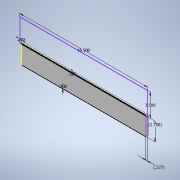
# Autodesk Inventor part: Part3
Saved by Autodesk Inventor 2021 (Build 250183000, 183)
## iProperties
Created: 2020-09-03
Part Number: Part3
Material: Generic
Document SubType Name: Modeling
Designer: deli
Density: 1 g/cm^3
Appearance: Default
Author: deli
Autodesk Inventor part; units mm, degrees
ref_plane "YZ Plane" through (0, 0, 0) normal (1, 0, 0) x (0, 1, 0)
ref_plane "XZ Plane" through (0, 0, 0) normal (0, 1, 0) x (-1, 0, 0)
ref_plane "XY Plane" through (0, 0, 0) normal (0, 0, 1) x (1, 0, 0)
sketch "Sketch1" plane through (0, 0, 0) normal (0, 0, 1) x (1, 0, 0)
  line L0 (-47.5672, 9.4536) -> (435.0328, 9.4536)
  line L1 (435.0328, 9.4536) -> (435.0328, -60.3964)
  line L2 (435.0328, -60.3964) -> (-47.5672, -60.3964)
  line L3 (-47.5672, -60.3964) -> (-47.5672, 9.4536)
  point P0 (0, 0)
  dimension "d0" = 482.6
  dimension "d1" = 69.85
  constraints: 8 end point, 2 parallel, 1 horizontal, 1 perpendicular
  measures "d0" distance of L1.end L2.end
  measures "d1" distance of L0.end L1.end
extrude "Extrusion1" add sketch "Sketch1" along normal blind 8.89
sketch "Sketch2" plane through (0, 0, 8.89) normal (0, 0, 1) x (1, 0, 0)
  line L0 (435.0328, 9.4536) -> (-47.5672, 9.4536) projected
  line L1 (-47.5672, 9.4536) -> (435.0328, 9.4536)
  line L2 (-48.1454, -60.3964) -> (435.0328, -60.3964)
  line L3 (435.0328, -60.3964) -> (435.0328, 12.6286)
  line L4 (435.0328, 12.6286) -> (-48.1454, 12.6286)
  line L5 (-48.1454, 12.6286) -> (-48.1454, -60.3964)
  line L6 (-47.5672, -60.3964) -> (435.0328, -60.3964) projected
  line L7 (-54.4954, 9.4536) -> (440.8046, 9.4536)
  line L8 (440.8046, 9.4536) -> (440.8046, 98.3536)
  line L9 (440.8046, 98.3536) -> (-54.4954, 98.3536)
  line L10 (-54.4954, 98.3536) -> (-54.4954, 9.4536)
  point P0 (0, 0)
  dimension "d6" = 0
  dimension "d7" = 3.175
  dimension "d8" = 495.3
  dimension "d9" = 88.9
  dimension "d10" = 6.35
  constraints: 18 end point, 4 parallel, 3 horizontal, 2 perpendicular
  measures "d6" distance between parallel lines of L6 L2
  measures "d7" distance between parallel lines of L4 L0
  measures "d8" distance of L9.end L8.end
  measures "d9" distance of L8.end L7.end
  measures "d10" distance between parallel lines of L5 L10
sketch "Sketch3" plane through (0, 0, 8.89) normal (0, 0, 1) x (1, 0, 0)
  line L0 (-47.5672, -60.3964) -> (435.0328, -60.3964) projected
  line L1 (435.0328, -60.3964) -> (435.0328, 9.4536) projected
  line L2 (435.0328, 9.4536) -> (-47.5672, 9.4536) projected
  line L3 (-47.5672, 9.4536) -> (-47.5672, -60.3964) projected
  line L4 (440.8046, 9.4536) -> (440.8046, 98.3536) projected
  line L5 (440.8046, 98.3536) -> (-54.4954, 98.3536) projected
  point P0 (0, 0)
  dimension "d11" = 5.7717
  dimension "d12" = 69.85
  measures "d11" distance between parallel lines of L4 L1
  measures "d12" vertical distance of L4.start L0.end
body "Solid1"
